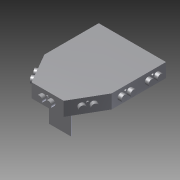
# Autodesk Inventor part: kepala 120 derajat
Saved by Autodesk Inventor 2012 (Build 160160000, 160)
## iProperties
Created: 2013-12-07
Part Number: kepala 120 derajat
Material: Default
Document SubType Name: Modeling
Designer: Irwan Haryanto
Density: 1 g/cm^3
Author: Irwan Haryanto
Autodesk Inventor part; units mm, degrees
ref_plane "YZ Plane" through (0, 0, 0) normal (1, 0, 0) x (0, 1, 0)
ref_plane "XZ Plane" through (0, 0, 0) normal (0, 1, 0) x (-1, 0, 0)
ref_plane "XY Plane" through (0, 0, 0) normal (0, 0, 1) x (1, 0, 0)
sketch "Sketch1" plane through (0, 0, 0) normal (0, 0, 1) x (1, 0, 0)
  line L0 (-41.7418, -140.2167) -> (41.7418, -140.2167)
  line L1 (41.7418, -140.2167) -> (87.255, -219.0478)
  line L2 (87.255, -219.0478) -> (87.255, -359.9816)
  line L3 (87.255, -359.9816) -> (-87.255, -359.9816)
  line L4 (-87.255, -359.9816) -> (-87.255, -219.0478)
  line L5 (-87.255, -219.0478) -> (-41.7418, -140.2167)
  point P0 (0, 0)
  dimension "d0" = 120
  dimension "d1" = 219.7649
  dimension "d2" = 174.51
  dimension "d3" = 120
  dimension "d4" = 150
  dimension "d5" = 150
  dimension "d6" = 91.0263
  dimension "d7" = 91.0263
  dimension "d8" = 83.4837
  dimension "d9" = 140.9338
  dimension "d10" = 140.9338
  constraints: 12 end point, 1 parallel, 1 perpendicular
  measures "d0" angle of L5 L0
  measures "d1" distance between parallel lines of L3 L0
  measures "d2" distance between parallel lines of L2 L4
  measures "d3" angle of L1 L0
  measures "d4" angle of L4 L5
  measures "d5" angle of L2 L1
  measures "d6" distance of L0.end L1.end
  measures "d7" distance of L4.end L0.start
  measures "d8" distance of L0.start L0.end
  measures "d9" distance of L3.end L4.end
  measures "d10" distance of L1.end L2.end
extrude "Extrusion1" add sketch "Sketch1" along normal blind 36
sketch "Sketch2" plane through (-41.7418, -140.2167, 0) normal (0, 1, 0) x (1, 0, 0)
  circle A0 centre (41.7418, -11.1) radius 2.95
  circle A1 centre (61.1168, -25.8) radius 1.5
  circle A2 centre (61.1168, -10.2) radius 1.5
  circle A3 centre (53.4418, -18) radius 8.25
  circle A4 centre (22.3668, -25.8) radius 1.5
  circle A5 centre (30.0418, -18) radius 8.25
  circle A6 centre (22.3668, -10.2) radius 1.5
  point P0 (41.7418, 0)
  dimension "d13" = 16.5
  dimension "d14" = 16.5
  dimension "d15" = 5.9
  dimension "d16" = 3
  dimension "d17" = 7.8
  dimension "d18" = 7.8
  dimension "d19" = 23.4
  dimension "d20" = 7.675
  dimension "d21" = 7.675
  dimension "d22" = 7.675
  dimension "d23" = 7.675
  dimension "d24" = 7.8
  dimension "d25" = 7.8
  dimension "d27" = 6.9
  constraints: 7 centre point
  measures "d13" diameter of A5
  measures "d14" diameter of A3
  measures "d15" diameter of A0
  measures "d16" diameter of A2
  measures "d17" vertical distance of A5.centre A6.centre
  measures "d18" vertical distance of A5.centre A4.centre
  measures "d19" distance of A3.centre A5.centre
  measures "d20" horizontal distance of A5.centre A6.centre
  measures "d21" horizontal distance of A5.centre A4.centre
  measures "d22" horizontal distance of A2.centre A3.centre
  measures "d23" horizontal distance of A1.centre A3.centre
  measures "d24" vertical distance of A3.centre A2.centre
  measures "d25" vertical distance of A3.centre A1.centre
  measures "d27" vertical distance of A0.centre A5.centre
extrude "Extrusion2" add sketch "Sketch2" along normal blind 10 contours A3 | A5
extrude "Extrusion3" add sketch "Sketch2" along normal blind 3 contours A0
sketch "Sketch3" plane through (87.255, -219.0478, 36) normal (0.8660254, 0.5, 0) x (0, 0, -1)
  circle A0 centre (25.8, 26.1382) radius 1.5
  circle A1 centre (18, 33.8132) radius 8.25
  circle A2 centre (10.2, 26.1382) radius 1.5
  circle A3 centre (24.9, 45.5132) radius 2.95
  circle A4 centre (18, 57.2132) radius 8.25
  circle A5 centre (10.2, 64.8882) radius 1.5
  circle A6 centre (25.8, 64.8882) radius 1.5
  point P0 (36, 233.3284)
  point P1 (18, 45.5132)
  point P2 (18, 45.5132)
  dimension "d49" = 16.5
  dimension "d50" = 16.5
  dimension "d51" = 5.9
  dimension "d52" = 3
  dimension "d53" = 7.675
  dimension "d54" = 7.675
  dimension "d55" = 23.4
  dimension "d56" = 7.8
  dimension "d57" = 7.8
  dimension "d58" = 7.8
  dimension "d59" = 7.8
  dimension "d60" = 7.675
  dimension "d61" = 7.675
  dimension "d62" = 11.7
  constraints: 7 centre point
  measures "d49" diameter of A4
  measures "d50" diameter of A1
  measures "d51" diameter of A3
  measures "d52" diameter of A0
  measures "d53" vertical distance of A4.centre A6.centre
  measures "d54" vertical distance of A4.centre A5.centre
  measures "d55" distance of A1.centre A4.centre
  measures "d56" horizontal distance of A4.centre A6.centre
  measures "d57" horizontal distance of A4.centre A5.centre
  measures "d58" horizontal distance of A0.centre A1.centre
  measures "d59" horizontal distance of A2.centre A1.centre
  measures "d60" vertical distance of A1.centre A0.centre
  measures "d61" vertical distance of A1.centre A2.centre
  measures "d62" vertical distance of A3.centre A4.centre
extrude "Extrusion4" add sketch "Sketch3" along normal blind 3 contours A3
extrude "Extrusion5" add sketch "Sketch3" along normal blind 10 contours A1 | A4
sketch "Sketch4" plane through (-41.7418, -140.2167, 0) normal (-0.8660254, 0.5, 0) x (0, 0, 1)
  circle A0 centre (11.1, -45.5132) radius 2.95
  circle A1 centre (25.8, -26.1382) radius 1.5
  circle A2 centre (10.2, -26.1382) radius 1.5
  circle A3 centre (18, -33.8132) radius 8.25
  circle A4 centre (25.8, -64.8882) radius 1.5
  circle A5 centre (18, -57.2132) radius 8.25
  circle A6 centre (10.2, -64.8882) radius 1.5
  point P0 (0, 142.3021)
  point P1 (18, -45.5132)
  point P2 (18, -45.5132)
  dimension "d67" = 16.5
  dimension "d68" = 16.5
  dimension "d69" = 5.9
  dimension "d70" = 3
  dimension "d71" = -7.675
  dimension "d72" = 7.675
  dimension "d73" = 23.4
  dimension "d74" = 7.8
  dimension "d75" = 7.8
  dimension "d76" = 7.8
  dimension "d77" = 7.8
  dimension "d78" = 7.675
  dimension "d79" = 7.675
  dimension "d80" = 6.9
  dimension "d81" = 11.7
  dimension "d82" = 6.9
  constraints: 7 centre point
  measures "d67" diameter of A5
  measures "d68" diameter of A3
  measures "d69" diameter of A0
  measures "d70" diameter of A2
  measures "d71" vertical distance of A5.centre A6.centre
  measures "d72" vertical distance of A5.centre A4.centre
  measures "d73" distance of A3.centre A5.centre
  measures "d74" horizontal distance of A5.centre A6.centre
  measures "d75" horizontal distance of A5.centre A4.centre
  measures "d76" horizontal distance of A2.centre A3.centre
  measures "d77" horizontal distance of A1.centre A3.centre
  measures "d78" vertical distance of A3.centre A2.centre
  measures "d79" vertical distance of A3.centre A1.centre
  measures "d80" horizontal distance of A5.centre A0.centre
  measures "d81" vertical distance of A0.centre A5.centre
  measures "d82" horizontal distance of A3.centre A0.centre
extrude "Extrusion6" add sketch "Sketch4" along normal blind 10 contours A3 | A5
extrude "Extrusion7" add sketch "Sketch4" along normal blind 3 contours A0
sketch "Sketch5" plane through (87.255, -359.9816, 0) normal (1, 0, 0) x (0, 0, -1)
  line L0 (-36, 140.9338) -> (-36, 0) projected
  line L1 (0, 140.9338) -> (0, 0) projected
  line L2 (0, 140.9338) -> (-36, 140.9338) projected
  circle A0 centre (-11.1, 105.7003) radius 2.95
  circle A1 centre (-25.8, 86.3253) radius 1.5
  circle A2 centre (-10.2, 86.3253) radius 1.5
  circle A3 centre (-18, 94.0003) radius 8.25
  circle A4 centre (-25.8, 125.0753) radius 1.5
  circle A5 centre (-18, 117.4003) radius 8.25
  circle A6 centre (-10.2, 125.0753) radius 1.5
  line L3 (-36, 70.4669) -> (0, 70.4669)
  circle A7 centre (-10.2, 54.6085) radius 1.5
  circle A8 centre (-18, 46.9335) radius 8.25
  circle A9 centre (-25.8, 54.6085) radius 1.5
  circle A10 centre (-11.1, 35.2335) radius 2.95
  circle A11 centre (-18, 23.5335) radius 8.25
  circle A12 centre (-25.8, 15.8585) radius 1.5
  circle A13 centre (-10.2, 15.8585) radius 1.5
  point P0 (0, 359.9816)
  point P1 (-18, 105.7003)
  point P2 (-18, 70.4669)
  point P3 (-18, 105.7003)
  point P4 (-18, 35.2335)
  point P5 (-18, 35.2335)
  dimension "d87" = 16.5
  dimension "d88" = 16.5
  dimension "d89" = 5.9
  dimension "d90" = 3
  dimension "d91" = 7.675
  dimension "d92" = 7.675
  dimension "d93" = 23.4
  dimension "d94" = 7.8
  dimension "d95" = 7.8
  dimension "d96" = 7.8
  dimension "d97" = 7.8
  dimension "d98" = 7.675
  dimension "d99" = 7.675
  dimension "d100" = 6.9
  dimension "d101" = 11.7
  dimension "d102" = 6.9
  dimension "d103" = 70.4669
  dimension "d104" = 35.2335
  constraints: 14 centre point, 9 symmetric about line, 2 end point, 2 midpoint, 7 other
  measures "d87" diameter of A5
  measures "d88" diameter of A3
  measures "d89" diameter of A0
  measures "d90" diameter of A2
  measures "d91" vertical distance of A5.centre A6.centre
  measures "d92" vertical distance of A5.centre A4.centre
  measures "d93" distance of A3.centre A5.centre
  measures "d94" horizontal distance of A5.centre A6.centre
  measures "d95" horizontal distance of A5.centre A4.centre
  measures "d96" horizontal distance of A2.centre A3.centre
  measures "d97" horizontal distance of A1.centre A3.centre
  measures "d98" vertical distance of A3.centre A2.centre
  measures "d99" vertical distance of A3.centre A1.centre
  measures "d100" horizontal distance of A5.centre A0.centre
  measures "d101" vertical distance of A0.centre A5.centre
  measures "d102" horizontal distance of A3.centre A0.centre
  measures "d103" distance between parallel lines of L3 L2
  measures "d104" distance from line of L2 point (-18, 105.7)
extrude "Extrusion8" add sketch "Sketch5" along normal blind 3 contours A0 | A10
extrude "Extrusion9" add sketch "Sketch5" along normal blind 10 contours A3 | A5 | A8 | A11
sketch "Sketch6" plane through (-87.255, -359.9816, 0) normal (0, -1, 0) x (1, 0, 0)
  line L0 (174.51, 36) -> (0, 36) projected
  line L1 (174.51, 0) -> (174.51, 36) projected
  line L2 (87.255, 0) -> (87.255, 36)
  circle A0 centre (111.5075, 10.2) radius 1.5
  circle A1 centre (119.1825, 18) radius 8.25
  circle A2 centre (111.5075, 25.8) radius 1.5
  circle A3 centre (130.8825, 11.1) radius 2.95
  circle A4 centre (142.5825, 18) radius 8.25
  circle A5 centre (150.2575, 25.8) radius 1.5
  circle A6 centre (150.2575, 10.2) radius 1.5
  circle A7 centre (43.6275, 11.1) radius 2.95
  circle A8 centre (55.3275, 18) radius 8.25
  circle A9 centre (63.0025, 25.8) radius 1.5
  circle A10 centre (63.0025, 10.2) radius 1.5
  circle A11 centre (24.2525, 10.2) radius 1.5
  circle A12 centre (31.9275, 18) radius 8.25
  circle A13 centre (24.2525, 25.8) radius 1.5
  point P0 (130.8825, 18)
  point P1 (130.8825, 18)
  point P2 (43.6275, 18)
  point P3 (43.6275, 18)
  dimension "d125" = 87.255
  dimension "d126" = 43.6275
  dimension "d127" = 16.5
  dimension "d128" = 16.5
  dimension "d129" = 5.9
  dimension "d130" = 3
  dimension "d131" = -7.8
  dimension "d132" = 7.8
  dimension "d133" = 23.4
  dimension "d134" = 7.675
  dimension "d135" = 7.675
  dimension "d136" = 7.675
  dimension "d137" = 7.675
  dimension "d138" = 7.8
  dimension "d139" = 7.8
  dimension "d140" = 11.7
  dimension "d141" = 6.9
  dimension "d142" = 11.7
  constraints: 14 centre point, 9 symmetric about line, 2 end point, 1 midpoint, 7 other
  measures "d125" distance between parallel lines of L2 L1
  measures "d126" distance from line of point (130.882, 18) L1
  measures "d127" diameter of A4
  measures "d128" diameter of A1
  measures "d129" diameter of A3
  measures "d130" diameter of A0
  measures "d131" vertical distance of A4.centre A6.centre
  measures "d132" vertical distance of A4.centre A5.centre
  measures "d133" distance of A1.centre A4.centre
  measures "d134" horizontal distance of A4.centre A6.centre
  measures "d135" horizontal distance of A4.centre A5.centre
  measures "d136" horizontal distance of A0.centre A1.centre
  measures "d137" horizontal distance of A2.centre A1.centre
  measures "d138" vertical distance of A1.centre A0.centre
  measures "d139" vertical distance of A1.centre A2.centre
  measures "d140" horizontal distance of A4.centre A3.centre
  measures "d141" vertical distance of A3.centre A4.centre
  measures "d142" horizontal distance of A1.centre A3.centre
extrude "Extrusion10" add sketch "Sketch6" along normal blind 10 contours A1 | A4 | A8 | A12
extrude "Extrusion11" add sketch "Sketch6" along normal blind 3 contours A3 | A7
sketch "Sketch7" plane through (-87.255, -359.9816, 0) normal (-1, 0, 0) x (0, 0, 1)
  line L0 (36, 0) -> (36, 140.9338) projected
  line L1 (0, 140.9338) -> (36, 140.9338) projected
  line L2 (0, 0) -> (0, 140.9338) projected
  line L3 (0, 0) -> (36, 0) projected
  point P0 (0, 359.9816)
sketch "Sketch8" plane through (-87.255, -359.9816, 0) normal (-1, 0, 0) x (0, 0, 1)
  line L0 (0, 140.9338) -> (0, 0)
  circle A0 centre (10.2, 54.6085) radius 1.5
  circle A1 centre (18, 46.9335) radius 8.25
  circle A2 centre (25.8, 54.6085) radius 1.5
  circle A3 centre (11.1, 35.2335) radius 2.95
  circle A4 centre (18, 23.5335) radius 8.25
  circle A5 centre (25.8, 15.8585) radius 1.5
  circle A6 centre (10.2, 15.8585) radius 1.5
  circle A7 centre (25.8, 86.3253) radius 1.5
  circle A8 centre (10.2, 86.3253) radius 1.5
  circle A9 centre (18, 94.0003) radius 8.25
  circle A10 centre (11.1, 105.7003) radius 2.95
  circle A11 centre (18, 117.4003) radius 8.25
  circle A12 centre (10.2, 125.0753) radius 1.5
  circle A13 centre (25.8, 125.0753) radius 1.5
  point P0 (0, 359.9816)
  point P1 (0, 359.9816)
  point P2 (18, 35.2335)
  point P3 (18, 70.4669)
  point P4 (18, 35.234)
  point P5 (18, 105.7003)
  point P6 (18, 105.7003)
  point P7 (18, 70.4669)
  dimension "d147" = 16.5
  dimension "d148" = 16.5
  dimension "d149" = 5.9
  dimension "d150" = 3
  dimension "d151" = -7.675
  dimension "d152" = 7.675
  dimension "d153" = 23.4
  dimension "d154" = 7.8
  dimension "d155" = 7.8
  dimension "d156" = 7.8
  dimension "d157" = 7.8
  dimension "d158" = 7.675
  dimension "d159" = 7.675
  dimension "d160" = 6.9
  dimension "d161" = 11.7
  dimension "d162" = 6.9
  constraints: 14 centre point, 2 end point
  measures "d147" diameter of A4
  measures "d148" diameter of A1
  measures "d149" diameter of A3
  measures "d150" diameter of A0
  measures "d151" vertical distance of A4.centre A6.centre
  measures "d152" vertical distance of A4.centre A5.centre
  measures "d153" distance of A1.centre A4.centre
  measures "d154" horizontal distance of A4.centre A6.centre
  measures "d155" horizontal distance of A4.centre A5.centre
  measures "d156" horizontal distance of A0.centre A1.centre
  measures "d157" horizontal distance of A2.centre A1.centre
  measures "d158" vertical distance of A1.centre A0.centre
  measures "d159" vertical distance of A1.centre A2.centre
  measures "d160" horizontal distance of A4.centre A3.centre
  measures "d161" vertical distance of A3.centre A4.centre
  measures "d162" horizontal distance of A1.centre A3.centre
extrude "Extrusion12" add sketch "Sketch8" along normal blind 3 contours A3 | A10
extrude "Extrusion13" add sketch "Sketch8" along normal blind 10 contours A1 | A4 | A9 | A11
sketch "Sketch9" plane through (0, 0, 36) normal (0, 0, 1) x (1, 0, 0)
  circle A0 centre (29.975, -290.0862) radius 1.5
  circle A1 centre (24.975, -295.2032) radius 1.5
  circle A2 centre (19.975, -300.2032) radius 1.5
  circle A3 centre (24.975, -305.2032) radius 1.5
  line L0 (7, -174.6532) -> (19, -174.6532)
  circle A4 centre (19.4208, -190.1532) radius 1.5
  circle A5 centre (19.4208, -200.1532) radius 1.5
  circle A6 centre (24.975, -195.1532) radius 1.5
  line L1 (87.255, -359.9367) -> (-87.255, -359.9367)
  circle A7 centre (-19.4208, -200.1532) radius 1.5
  circle A8 centre (-19.4208, -190.1532) radius 1.5
  circle A9 centre (-24.975, -305.2032) radius 1.5
  circle A10 centre (-24.975, -295.2032) radius 1.5
  circle A11 centre (-29.975, -290.0862) radius 1.5
  circle A12 centre (-19.975, -300.2032) radius 1.5
  circle A13 centre (24.975, -205.1532) radius 1.5
  circle A14 centre (29.975, -210.2702) radius 1.5
  circle A15 centre (-24.975, -205.1532) radius 1.5
  circle A16 centre (-29.975, -210.2702) radius 1.5
  circle A17 centre (-24.975, -195.1532) radius 1.5
  line L2 (19, -174.6532) -> (7, -174.6532)
  line L3 (87.255, -359.9367) -> (-87.255, -359.9367)
  line L4 (0, -172.6532) -> (0, -174.6532)
  line L5 (0, -174.6532) -> (-28.5, -174.6532)
  line L6 (0, -174.6532) -> (28.5, -174.6532)
  line L7 (-28.5, -174.6532) -> (-28.5, -172.6532)
  line L8 (-28.5, -172.6532) -> (28.5, -172.6532)
  line L9 (28.5, -174.6532) -> (28.5, -172.6532)
  point P0 (0, 0)
  dimension "d201" = 3
  dimension "d202" = 3
  dimension "d203" = 3
  dimension "d204" = 3
  dimension "d205" = 3
  dimension "d206" = -5.117
  dimension "d207" = 10
  dimension "d208" = 15.117
  dimension "d209" = 10
  dimension "d210" = 5.5542
  dimension "d211" = 5
  dimension "d212" = 5
  dimension "d213" = 5.5542
  dimension "d214" = 5.5542
  dimension "d215" = 5
  dimension "d216" = 5
  dimension "d217" = 3
  dimension "d218" = 3
  dimension "d219" = 3
  dimension "d220" = 5.117
  dimension "d221" = 0
  dimension "d222" = 15.117
  dimension "d223" = 3
  dimension "d224" = 5
  dimension "d225" = 5
  dimension "d226" = 5
  dimension "d227" = 5
  dimension "d228" = 5
  dimension "d251" = 28.5
  dimension "d252" = 28.5
  dimension "d253" = 2
  constraints: 20 end point, 18 centre point, 4 perpendicular, 1 midpoint, 1 point on line
  measures "d201" diameter of A14
  measures "d202" diameter of A13
  measures "d203" diameter of A6
  measures "d204" diameter of A5
  measures "d205" diameter of A4
  measures "d206" vertical distance of A13.centre A14.centre
  measures "d207" distance of A13.centre A6.centre
  measures "d208" vertical distance of A14.centre A6.centre
  measures "d209" distance of A5.centre A4.centre
  measures "d210" horizontal distance of A5.centre A6.centre
  measures "d211" vertical distance of A6.centre A4.centre
  measures "d212" vertical distance of A5.centre A6.centre
  measures "d213" horizontal distance of A6.centre A4.centre
  measures "d214" horizontal distance of A13.centre A5.centre
  measures "d215" vertical distance of A13.centre A5.centre
  measures "d216" horizontal distance of A14.centre A13.centre
  measures "d217" diameter of A1
  measures "d218" diameter of A3
  measures "d219" diameter of A0
  measures "d220" vertical distance of A1.centre A0.centre
  measures "d221" horizontal distance of A3.centre A1.centre
  measures "d222" vertical distance of A3.centre A0.centre
  measures "d223" diameter of A2
  measures "d224" horizontal distance of A2.centre A1.centre
  measures "d225" horizontal distance of A2.centre A1.centre
  measures "d226" horizontal distance of A2.centre A3.centre
  measures "d227" horizontal distance of A3.centre A2.centre
  measures "d228" horizontal distance of A1.centre A0.centre
  measures "d251" distance of L4.end L5.end
  measures "d252" distance of L4.end L6.end
  measures "d253" distance of L5.end L7.end
extrude "Extrusion14" add sketch "Sketch9" along normal blind 67 contours L6 L4 L8 L9 L0 | L5 L7 L8 L4
sketch "Sketch10" plane through (0, 0, 36) normal (0, 0, 1) x (1, 0, 0)
  line L0 (7, -174.6532) -> (19, -174.6532)
  line L1 (19, -174.6532) -> (7, -174.6532)
  circle A0 centre (-19.4208, -190.1532) radius 1.5
  circle A1 centre (-24.975, -195.1532) radius 1.5
  circle A2 centre (19.4208, -200.1532) radius 1.5
  circle A3 centre (-19.4208, -200.1532) radius 1.5
  circle A4 centre (-29.975, -210.2702) radius 1.5
  circle A5 centre (-24.975, -205.1532) radius 1.5
  circle A6 centre (19.4208, -190.1532) radius 1.5
  circle A7 centre (24.975, -195.1532) radius 1.5
  circle A8 centre (24.975, -205.1532) radius 1.5
  circle A9 centre (29.975, -210.2702) radius 1.5
  circle A10 centre (29.975, -290.0862) radius 1.5
  circle A11 centre (24.975, -295.2032) radius 1.5
  circle A12 centre (19.975, -300.2032) radius 1.5
  circle A13 centre (24.975, -305.2032) radius 1.5
  circle A14 centre (-24.975, -305.2032) radius 1.5
  circle A15 centre (-19.975, -300.2032) radius 1.5
  line L2 (87.255, -359.9367) -> (-87.255, -359.9367)
  line L3 (87.255, -359.9367) -> (-87.255, -359.9367)
  circle A16 centre (-24.975, -295.2032) radius 1.5
  circle A17 centre (-29.975, -290.0862) radius 1.5
  line L4 (0, -172.6532) -> (0, -174.6532)
  line L5 (0, -174.6532) -> (-28.5, -174.6532)
  line L6 (0, -174.6532) -> (28.5, -174.6532)
  line L7 (-28.5, -174.6532) -> (-28.5, -172.6532)
  line L8 (-28.5, -172.6532) -> (28.5, -172.6532)
  line L9 (28.5, -174.6532) -> (28.5, -172.6532)
  point P0 (0, 0)
  point P1 (0, 0)
  dimension "d256" = 3
  dimension "d257" = 3
  dimension "d258" = 3
  dimension "d259" = 3
  dimension "d260" = 3
  dimension "d261" = -5.117
  dimension "d262" = 10
  dimension "d263" = 15.117
  dimension "d264" = 10
  dimension "d265" = 5.5542
  dimension "d266" = 5
  dimension "d267" = 5
  dimension "d268" = 5.5542
  dimension "d269" = 5.5542
  dimension "d270" = 5
  dimension "d271" = 5
  dimension "d272" = 3
  dimension "d273" = 3
  dimension "d274" = 3
  dimension "d275" = 5.117
  dimension "d276" = 0
  dimension "d277" = 15.117
  dimension "d278" = 3
  dimension "d279" = 5
  dimension "d280" = 5
  dimension "d281" = 5
  dimension "d282" = 5
  dimension "d283" = 5
  dimension "d284" = 28.5
  dimension "d285" = 28.5
  dimension "d286" = 2
  constraints: 20 end point, 18 centre point, 4 perpendicular, 1 midpoint, 1 point on line
  measures "d256" diameter of A9
  measures "d257" diameter of A8
  measures "d258" diameter of A7
  measures "d259" diameter of A2
  measures "d260" diameter of A6
  measures "d261" vertical distance of A8.centre A9.centre
  measures "d262" distance of A8.centre A7.centre
  measures "d263" vertical distance of A9.centre A7.centre
  measures "d264" distance of A2.centre A6.centre
  measures "d265" horizontal distance of A2.centre A7.centre
  measures "d266" vertical distance of A7.centre A6.centre
  measures "d267" vertical distance of A2.centre A7.centre
  measures "d268" horizontal distance of A7.centre A6.centre
  measures "d269" horizontal distance of A8.centre A2.centre
  measures "d270" vertical distance of A8.centre A2.centre
  measures "d271" horizontal distance of A9.centre A8.centre
  measures "d272" diameter of A11
  measures "d273" diameter of A13
  measures "d274" diameter of A10
  measures "d275" vertical distance of A11.centre A10.centre
  measures "d276" horizontal distance of A13.centre A11.centre
  measures "d277" vertical distance of A13.centre A10.centre
  measures "d278" diameter of A12
  measures "d279" horizontal distance of A12.centre A11.centre
  measures "d280" horizontal distance of A12.centre A11.centre
  measures "d281" horizontal distance of A12.centre A13.centre
  measures "d282" horizontal distance of A13.centre A12.centre
  measures "d283" horizontal distance of A11.centre A10.centre
  measures "d284" distance of L4.end L5.end
  measures "d285" distance of L4.end L6.end
  measures "d286" distance of L5.end L7.end
hole "Hole1" at (-19.4208, -190.1532, 36) at (-24.975, -195.1532, 36) at (-19.4208, -200.1532, 36) at (-24.975, -205.1532, 36) at (-29.975, -210.2702, 36) at (19.4208, -190.1532, 36) at (24.975, -195.1532, 36) at (19.4208, -200.1532, 36) at (29.975, -210.2702, 36) at (24.975, -205.1532, 36) at (29.975, -290.0862, 36) at (24.975, -295.2032, 36) at (19.975, -300.2032, 36) at (24.975, -305.2032, 36) at (-24.975, -305.2032, 36) at (-19.975, -300.2032, 36) at (-24.975, -295.2032, 36) at (-29.975, -290.0862, 36) direction (0, 0, -1) diameter 3 depth 10 tip angle 118
body "Solid1"
